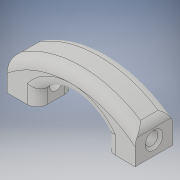
# Autodesk Inventor part: cable clamp
Saved by Autodesk Inventor 2019 (Build 230136000, 136)
## iProperties
Created: 2019-05-24
Part Number: cable clamp
Material: Generic
Document SubType Name: Modeling
Designer: Ironic
Density: 1 g/cm^3
Appearance: Default
Author: Ironic
Autodesk Inventor part; units mm, degrees
ref_plane "YZ Plane" through (0, 0, 0) normal (1, 0, 0) x (0, 1, 0)
ref_plane "XZ Plane" through (0, 0, 0) normal (0, 1, 0) x (-1, 0, 0)
ref_plane "XY Plane" through (0, 0, 0) normal (0, 0, 1) x (1, 0, 0)
sketch "Sketch1" plane through (0, 0, 0) normal (0, 0, 1) x (1, 0, 0)
  line L0 (-12.75, -5) -> (12.75, -5)
  line L1 (12.75, -5) -> (12.75, 5)
  line L2 (12.75, 5) -> (-12.75, 5)
  line L3 (-12.75, 5) -> (-12.75, -5)
  line L4 (-12.75, -5) -> (12.75, 5) construction
  line L5 (12.75, -5) -> (-12.75, 5) construction
  arc A0 (0, 1) -> (-8.462442, -5) centre (0.022849, -7.999971) ccw
  arc A1 (8.508141, -5) -> (0, 1) centre (0.022849, -7.999971) ccw
  arc A2 (12.75, 0.928678) -> (-12.75, 0.913128) centre (0.010933, -17.00777) ccw
  line L6 (-6.75, -2.07304) -> (-6.75, -5)
  line L7 (6.795698, -2.07304) -> (6.795698, -5)
  point P0 (0, 0)
  dimension "d0" = 25.5
  dimension "d1" = 10
  dimension "d2" = 6
  dimension "d3" = 9
  dimension "d15" = 6
  constraints: 16 end point, 8 point on circle, 6 point on line, 3 centre point, 3 perpendicular, 2 midpoint, 2 parallel, 1 coincident, 1 horizontal
  measures "d0" distance of L2.end L1.end
  measures "d1" distance of L1.end L0.end
  measures "d2" distance from line of L0 A0.start
  measures "d3" radius of A0
  measures "d15" distance between parallel lines of L3 L6
sketch "Sketch1 outline for Extrusion1" plane through (0, 0, 0) normal (0, 0, 1) x (1, 0, 0)
  line L0 (-6.75, -5) -> (-6.75, -2.07304)
  arc A0 (-6.75, -2.07304) -> (6.795698, -2.07304) centre (0.022849, -7.999971) cw
  line L1 (6.795698, -2.07304) -> (6.795698, -5)
  line L2 (6.795698, -5) -> (12.75, -5)
  line L3 (12.75, -5) -> (12.75, 0.928678)
  arc A1 (12.75, 0.928678) -> (-12.75, 0.913128) centre (0.010933, -17.00777) ccw
  line L4 (-12.75, 0.913128) -> (-12.75, -5)
  line L5 (-12.75, -5) -> (-6.75, -5)
extrude "Extrusion1" add sketch "Sketch1 outline for Extrusion1" along normal mid plane 7.5
sketch "Sketch2" plane through (-12.75, -5, 3.75) normal (-1, 0, 0) x (0, 0, 1)
  circle A0 centre (-3.75, 2.75) radius 1.25
  line L0 (0, 0) -> (-7.5, 0) projected
  point P0 (-3.75, 5)
  dimension "d6" = 2.5
  dimension "d7" = 2.75
  constraints: 1 centre point
  measures "d6" diameter of A0
  measures "d7" distance from line of L0 A0.centre
sketch "Sketch2 outline for Extrusion2" plane through (-12.75, -5, 3.75) normal (-1, 0, 0) x (0, 0, 1)
  circle A0 centre (-3.75, 2.75) radius 1.25
extrude "Extrusion2" cut sketch "Sketch2 outline for Extrusion2" against normal through all
fillet "Fillet1" radius 2 10 edges at (0.0228, 1, 3.75) (0.0228, 1, -3.75) (-0.0025, 4.9922, 3.75) (-0.0025, 4.9922, -3.75) (12.75, 0.9287, 0) (-12.75, 0.9131, 0) (-6.75, -3.5365, 3.75) (-6.75, -3.5365, -3.75) (6.7957, -3.5365, 3.75) (6.7957, -3.5365, -3.75)
chamfer "Chamfer1" distance 0.5 angle 45 2 edges at (-12.75, -2.25, -1.25) (12.75, -2.25, -1.25)
body "Solid1"
